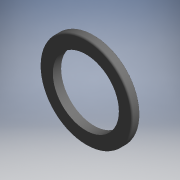
# Autodesk Inventor part: LZ80_Dichtring
Saved by Autodesk Inventor 2021 (Build 250183000, 183)
## iProperties
Part Number: LZ80_Dichtring
Material: Generic
Catalog Web Link: www.cadenas.de
Description: LZ80 Dichtring-Bauteil LZ80
Vendor: ROSEKRIEGER
Document SubType Name: Modeling
Designer: partserver
Manufacturer: ROSEKRIEGER
Mass: 5.95695 g
Surface Area: 37.688 cm^2
Volume: 5.95695 cm^3
Density: 1 g/cm^3
Appearance: PSOLRGB-128-128-128
Category: PARTsolutions
Company: ROSEKRIEGER
PSOL_IDENT_0: {$CADENAS_DATA\23d-libs\rose_krieger\linearkomponenten\pool_lineartechnik\_hubsaeule_zyliinder\elekt
PSOL_IDENT_1: rozylinder\elekzyl_lz80\lz80_dichtring.prj},167 {VTYP=3D},{NB=LZ80_Dichtring},{LINA=LZ80_Dichtring},
PSOL_IDENT_2: {NN=LZ80 Dichtring},{DATE=12.11.2020 14:43:35},{GEOMDATE=30.11.2006},{VERSION=},{LINEID=10},{WBVAR=}
PSOL_IDENT_3: ,{WBNUMERIC=}  {NB=LZ80_Dichtring},{LINA=LZ80_Dichtring},{KT=DUMMY},{IDNR=},{ARTIKEL=LZ80_Dichtring}
PSOL_IDENT_4: ,{AUSDURCH=56.000},{INDURCH=40.000},{HOEHE=5.000},{RADIUS=1.000}
NB: LZ80_Dichtring
NN: LZ80 Dichtring
NT: Bauteil LZ80
NBSYN: $ARTIKEL.
LINA: LZ80_Dichtring
CATALOG: RK Rose+Krieger
ARTIKEL: LZ80_Dichtring
AUSDURCH: 56
INDURCH: 40
HOEHE: 5
RADIUS: 1
SUPPLIER: ROSEKRIEGER
ARTICLENO: LZ80_Dichtring
BOMINFO: LZ80_Dichtring
CREATOR: CADENAS GmbH
Title: LZ80_Dichtring
Author: Cadenas PARTsolutions
Comments: Bauteil LZ80
Autodesk Inventor part; units mm, degrees
sketch "Skizze_1" plane through (0, 0, 0) normal (0, 0, 1) x (1, 0, 0)
  line L0 (0, -50) -> (0, 50)
  line L1 (20, 0) -> (20, -5)
  line L2 (20, -5) -> (27, -5)
  arc A0 (27, -5) -> (28, -4) centre (27, -4) ccw
  line L3 (28, -4) -> (28, -1)
  arc A1 (28, -1) -> (27, 0) centre (27, -1) ccw
  line L4 (27, 0) -> (20, 0)
  constraints: 10 end point, 4 point on circle, 2 centre point
revolve "Revolution1" add sketch "Skizze_1" angle 360 about axis through (0, -50, 0) along (0, -1, 0)
ref_plane "EPRING_XY" through (0, 0, 0) normal (0, 1, 0) x (1, 0, 0)
ref_plane "EPRING_YZ" through (0, 0, 0) normal (1, 0, 0) x (0, 0, -1)
ref_plane "EPRING_ZX" through (0, 0, 0) normal (0, 0, -1) x (0, 1, 0)
body "Solid1"
